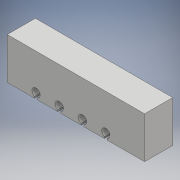
# Autodesk Inventor part: Lateral
Saved by Autodesk Inventor 2017 (Build 210142000, 142)
## iProperties
Created: 2021-02-12
Part Number: Lateral
Material: Generic
Document SubType Name: Modeling
Designer: USUARIO
Density: 1 g/cm^3
Appearance: Default
Author: USUARIO
Autodesk Inventor part; units mm, degrees
ref_plane "YZ Plane" through (0, 0, 0) normal (1, 0, 0) x (0, 1, 0)
ref_plane "XZ Plane" through (0, 0, 0) normal (0, 1, 0) x (-1, 0, 0)
ref_plane "XY Plane" through (0, 0, 0) normal (0, 0, 1) x (1, 0, 0)
sketch "Sketch1" plane through (0, 0, 0) normal (0, 1, 0) x (-1, 0, 0)
  line L0 (0, 0) -> (248, 0)
  line L1 (248, 0) -> (248, -75)
  line L2 (248, -75) -> (0, -75)
  line L3 (0, -75) -> (0, 0)
  dimension "d0" = 248
  dimension "d1" = 75
  constraints: 8 end point, 2 parallel, 1 horizontal, 1 perpendicular
  measures "d0" distance of L1.end L2.end
  measures "d1" distance of L0.end L1.end
extrude "Extrusion1" add sketch "Sketch1" along normal blind 50.8
sketch "Sketch2" plane through (0, 50.8, 0) normal (0, 1, 0) x (1, 0, 0)
  circle A0 centre (-196, 65) radius 7.5
  line L0 (0, 75) -> (-248, 75) projected
  line L1 (-248, 75) -> (-248, 0) projected
  circle A1 centre (-154, 65) radius 7.5
  circle A2 centre (-112, 65) radius 7.5
  circle A3 centre (-70, 65) radius 7.5
  point P0 (0, 0)
  dimension "d4" = 15
  dimension "d5" = 10
  dimension "d6" = 52
  dimension "d12" = 42
  constraints: 4 centre point, 1 horizontal, 6 other
  measures "d4" diameter of A0
  measures "d5" distance from line of A0.centre L0
  measures "d6" distance from line of A0.centre L1
  measures "d12" distance of A0.centre A1.centre
extrude "Extrusion2" cut sketch "Sketch2" against normal blind 50.8
sketch "Sketch3" plane through (0, 50.8, 0) normal (0, 1, 0) x (1, 0, 0)
  line L0 (0, 75) -> (-248, 75) projected
  line L1 (-198.5, 75) -> (-193.5, 75)
  line L2 (-193.5, 75) -> (-193.5, 72)
  line L3 (-193.5, 72) -> (-198.5, 72)
  line L4 (-198.5, 72) -> (-198.5, 75)
  circle A0 centre (-196, 65) radius 7.5 projected
  line L5 (-151.5, 75) -> (-151.5, 72)
  line L6 (-151.5, 72) -> (-156.5, 72)
  line L7 (-156.5, 72) -> (-156.5, 75)
  line L8 (-156.5, 75) -> (-151.5, 75)
  line L9 (-109.5, 75) -> (-109.5, 72)
  line L10 (-109.5, 72) -> (-114.5, 72)
  line L11 (-114.5, 72) -> (-114.5, 75)
  line L12 (-114.5, 75) -> (-109.5, 75)
  line L13 (-67.5, 75) -> (-67.5, 72)
  line L14 (-67.5, 72) -> (-72.5, 72)
  line L15 (-72.5, 72) -> (-72.5, 75)
  line L16 (-72.5, 75) -> (-67.5, 75)
  point P0 (0, 0)
  dimension "d16" = 5
  dimension "d17" = 3
  dimension "d18" = 2.5
  dimension "d24" = 42
  constraints: 32 end point, 2 horizontal, 2 parallel, 1 perpendicular, 1 point on line, 24 other
  measures "d16" distance of L2.end L3.end
  measures "d17" distance of L1.end L2.end
  measures "d18" distance from line of L4 A0.centre
  measures "d24" distance of L1.end L5.start
extrude "Extrusion3" cut sketch "Sketch3" against normal blind 50.8 contours L13 L14 L15 L0 | L2 A0 L4 L0 | L5 L6 L7 L0 | L9 L10 L11 L0 | L2 L3 L4 A0 picked at (-196.2826, 72.1506)
body "Solid1"
